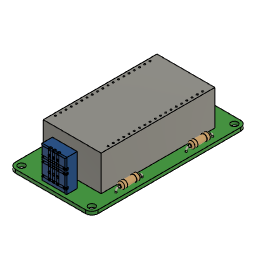
Gr3 3D v1 (Autodesk Fusion 360 archive; units mm, degrees)
design "PCB_PDP"
Autodesk Fusion 360 part; units mm, degrees
note: some values were not read from the file. Set by a fixed rule: which face or edge a step refers to.
sketch "Sketch1" plane through (0, 0, 0) normal (0, 0, 1) x (1, 0, 0)
  line L0 (0, 0) -> (79, 0)
  line L1 (79, 0) -> (79, 44)
  line L2 (79, 44) -> (0, 44)
  line L3 (0, 44) -> (0, 0)
  dimension "d1" = 79
  dimension "d2" = 44
  constraint horizontal L0
  constraint vertical L1
  constraint horizontal L2
  constraint vertical L3
  constraint coincident L0.start L3.end
  measures "d1" distance of L0.start L0.end
  measures "d2" distance of L0.start L2.end
extrude "Extrude1" add sketch "Sketch1" along normal blind 15 makes body 1
shell "Shell1" thickness 1.2 removed faces 1 at (26.3333, 29.3333, 15) on bodies 1
sketch "Sketch7" plane through (0, 0, 1.2) normal (0, 0, 1) x (-1, 0, 0)
  line L0 (-1.2, -42.8) -> (-1.2, -1.2)
  line L1 (-1.2, -1.2) -> (-77.8, -1.2)
  line L2 (-77.8, -1.2) -> (-77.8, -42.8)
  line L3 (-77.8, -42.8) -> (-1.2, -42.8)
  line L4 (-8.3254, -5.15) -> (-6.7377, -7.9)
  line L5 (-6.7377, -7.9) -> (-3.5623, -7.9)
  line L6 (-3.5623, -7.9) -> (-1.9746, -5.15)
  line L7 (-1.9746, -5.15) -> (-3.5623, -2.4)
  line L8 (-3.5623, -2.4) -> (-6.7377, -2.4)
  line L9 (-6.7377, -2.4) -> (-8.3254, -5.15)
  line L10 (-2, -42) -> (-77, -42) construction
  line L11 (-77, -42) -> (-77, -2) construction
  line L12 (-77, -2) -> (-2, -2) construction
  line L13 (-2, -2) -> (-2, -42) construction
  line L14 (-77, -42) -> (-2, -2) construction
  line L15 (-1.2, -42.8) -> (-77.8, -1.2) construction
  line L16 (-7.1996, -8.7) -> (-3.1004, -8.7)
  line L17 (-3.1004, -8.7) -> (-1.0508, -5.15)
  line L18 (-1.0508, -5.15) -> (-3.1004, -1.6)
  line L19 (-3.1004, -1.6) -> (-7.1996, -1.6)
  line L20 (-7.1996, -1.6) -> (-9.2492, -5.15)
  line L21 (-9.2492, -5.15) -> (-7.1996, -8.7)
  circle A0 centre (-5.15, -38.85) radius 3.3
  circle A1 centre (-73.85, -5.15) radius 3.3
  line L22 (-72.2623, -36.1) -> (-75.4377, -36.1)
  line L23 (-75.4377, -36.1) -> (-77.0254, -38.85)
  line L24 (-77.0254, -38.85) -> (-75.4377, -41.6)
  line L25 (-75.4377, -41.6) -> (-72.2623, -41.6)
  line L26 (-72.2623, -41.6) -> (-70.6746, -38.85)
  line L27 (-70.6746, -38.85) -> (-72.2623, -36.1)
  line L28 (-69.7508, -38.85) -> (-71.8004, -35.3)
  line L29 (-71.8004, -35.3) -> (-75.8996, -35.3)
  line L30 (-75.8996, -35.3) -> (-77.9492, -38.85)
  line L31 (-77.9492, -38.85) -> (-75.8996, -42.4)
  line L32 (-75.8996, -42.4) -> (-71.8004, -42.4)
  line L33 (-71.8004, -42.4) -> (-69.7508, -38.85)
  circle A2 centre (-73.85, -38.85) radius 1.55
  circle A3 centre (-5.15, -5.15) radius 1.55
  point P0 (-5.15, -5.15)
  point P1 (-5.15, -5.15)
  point P2 (-73.85, -38.85)
  point P3 (-73.85, -38.85)
  dimension "d63" = 5.5
  dimension "d64" = 75
  dimension "d65" = 40
  dimension "d66" = 3.15
  dimension "d67" = 3.15
  dimension "d68" = 0.8
  dimension "d70" = 3.15
  dimension "d71" = 3.15
  dimension "d72" = 6.6
  dimension "d73" = 6.6
  dimension "d74" = 3.15
  dimension "d75" = 3.15
  dimension "d76" = 5.5
  dimension "d77" = 3.15
  dimension "d78" = 3.15
  dimension "d79" = 0.8
  dimension "d80" = 3.1
  dimension "d81" = 3.1
  constraint horizontal L5
  constraint horizontal L10
  constraint vertical L11
  constraint horizontal L12
  constraint vertical L13
  constraint coincident L0.start L3.end
  constraint coincident L1.end L2.start
  constraint midpoint L14 L15
  constraint coincident P1 P0
  constraint horizontal L16
  constraint horizontal L25
  constraint coincident P3 P2
  constraint horizontal L32
  measures "d63" distance of L6 L9
  measures "d64" distance of L10.start L10.end
  measures "d65" distance of L10.start L12.end
  measures "d66" distance of P1 L12
  measures "d67" distance of P1 L13
  measures "d68" distance of L4 L21
  measures "d70" distance of L10 A0.centre
  measures "d71" distance of L13 A0.centre
  measures "d72" diameter of A0
  measures "d73" diameter of A1
  measures "d74" distance of L12 A1.centre
  measures "d75" distance of L11 A1.centre
  measures "d76" distance of L23 L26
  measures "d77" distance of L10 P3
  measures "d78" distance of L11 P3
  measures "d79" distance of L26 L33
  measures "d80" diameter of A2
  measures "d81" diameter of A3
extrude "Extrude25" cut sketch "Sketch7" against normal blind 4 contours L4 L5 L6 L7 L8 L9 | L22 L23 L24 L25 L26 L27 | A3 bodies 1 makes body 2 at (75.0374, 39.8463, 0.4)
extrude "Extrude26" cut 1 faces at (74.3155, 38.9202, 1.2) along direction (0, 0, -1) blind 7 on bodies 2 bodies 2
extrude "Extrude27" add sketch "Sketch7" along normal blind 1.4 contours L0 L16 L17 L18 L19 L20 L21 | L2 L28 L29 L30 L31 L32 L33 bodies 1 2
extrude "Extrude28" add sketch "Sketch7" along normal blind 3.6 contours A0 | A1 bodies 1
extrude "Extrude29" add sketch "Sketch7" along normal blind 3.6 from surface at 1.4 separate body contours L4 L5 L6 L7 L8 L9 | L22 L23 L24 L25 L26 L27 makes body 3 at (3.6019, 5.2273, 5) makes body 4 at (75.0374, 39.8463, 5)
extrude "Extrude30" add 2 faces at (73.3208, 42.1333, 2.6) (8.2581, 6.3333, 2.6) along direction (0, 0, 1) blind 0.4 on bodies 1 bodies 1 3 4
sketch "Sketch8" plane through (0, 44, 0) normal (0, 1, 0) x (-1, 0, 0)
  line L0 (-79, 0) -> (0, 0)
  line L1 (0, 0) -> (0, 15)
  line L2 (0, 15) -> (-79, 15)
  line L3 (-79, 15) -> (-79, 0)
  line L4 (-76.989, 1.4627) -> (-6.2495, 1.4627) construction
  line L5 (-6.2495, 1.4627) -> (-6.2495, 12.898) construction
  line L6 (-6.2495, 12.898) -> (-76.989, 12.898) construction
  line L7 (-76.989, 12.898) -> (-76.989, 1.4627) construction
  line L8 (-3.0583, 1.7286) -> (-3.0583, 13.6958) construction
  line L9 (-3.0583, 13.6958) -> (-10.7705, 13.6958) construction
  line L10 (-10.7705, 13.6958) -> (-10.7705, 1.7286) construction
  line L11 (-10.7705, 1.7286) -> (-3.0583, 1.7286) construction
  dimension "d114" = 8
  dimension "d115" = 8
  text T0 "TD 2  GR03" font "Arial" height 8 align left top in box 70.7394 x 11.4353 at (-76.989, 1.4627) x (1, 0) y (0, 1) spacing 1 kerned
  text T1 "8>" font "Arial" height 8 align left top in box 11.9672 x 7.7122 at (-3.0583, 1.7286) x (0, 1) y (-1, 0) spacing 1 kerned
extrude "Extrude31" cut sketch "Sketch8" against normal blind 0.4 text T0 T1 bodies 1
extrude "Extrude32" add 1 faces at (8.2581, 6.3333, 3) along direction (0, 0, 1) blind 0.4 on bodies 1 bodies 1
extrude "Extrude33" cut 1 faces at (5.1114, 7.4986, 2.6) along direction (0, 0, 1) blind 0.4 on bodies 1 bodies 1
extrude "Extrude34" add 1 faces at (73.3208, 42.1333, 3) along direction (0, 0, 1) blind 0.4 on bodies 1 bodies 1
extrude "Extrude35" cut 1 faces at (73.8886, 41.1986, 2.6) along direction (0, 0, 1) blind 0.4 on bodies 1 bodies 1
extrude "Extrude36" cut 1 faces at (73.8886, 41.1986, 6.2) along direction (0, 0, -1) blind 1.4 on bodies 1 bodies 1
extrude "Extrude37" cut 1 faces at (5.1114, 7.4986, 6.2) along direction (0, 0, -1) blind 1.4 on bodies 1 bodies 1
extrude "Extrude38" add 1 faces at (5.2123, 2.8038, 3) along direction (0, 0, -1) blind 0.4 on bodies 1 bodies 1
extrude "Extrude39" add 1 faces at (73.9123, 41.1962, 3) along direction (0, 0, -1) blind 0.4 on bodies 1 bodies 1
extrude "Extrude40" cut 1 faces at (26.7333, 43.6, 15) along direction (0, 0, -1) blind 8.6 on bodies 1 bodies 1
extrude "Extrude41" add 1 faces at (52.2667, 0.4, 6.4) along direction (0, 0, 1) blind 0.1 on bodies 1 bodies 1

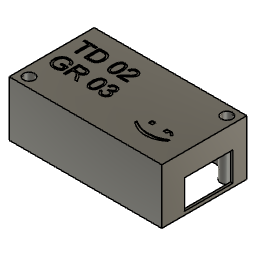
design "Haut"
Autodesk Fusion 360 part; units mm, degrees
sketch "Sketch1" plane through (0, 0, 0) normal (0, 0, 1) x (1, 0, 0)
  line L0 (0, 0) -> (79, 0)
  line L1 (79, 0) -> (79, 44)
  line L2 (79, 44) -> (0, 44)
  line L3 (0, 44) -> (0, 0)
  dimension "d1" = 79
  dimension "d2" = 44
  constraint horizontal L0
  constraint vertical L1
  constraint horizontal L2
  constraint vertical L3
  constraint coincident L0.start L3.end
  measures "d1" distance of L0.start L0.end
  measures "d2" distance of L0.start L2.end
extrude "Extrude1" add sketch "Sketch1" along normal blind 20
shell "Shell1" thickness 1.2 removed faces 1 at (26.3333, 29.3333, 0)
sketch "Sketch2" plane through (0, 0, 18.8) normal (0, 0, -1) x (1, 0, 0)
  line L0 (1.2, -1.2) -> (1.2, -42.8)
  line L1 (1.2, -42.8) -> (77.8, -42.8)
  line L2 (77.8, -42.8) -> (77.8, -1.2)
  line L3 (77.8, -1.2) -> (1.2, -1.2)
  line L4 (1.2, -1.2) -> (77.8, -42.8) construction
  line L5 (2, -2) -> (77, -2)
  line L6 (77, -2) -> (77, -42)
  line L7 (77, -42) -> (2, -42)
  line L8 (2, -42) -> (2, -2)
  line L9 (2, -42) -> (77, -2) construction
  circle A0 centre (5.15, -5.15) radius 1.55
  circle A1 centre (5.15, -5.15) radius 2.9
  circle A2 centre (5.15, -5.15) radius 3.3
  circle A3 centre (73.85, -38.85) radius 1.55
  circle A4 centre (73.85, -38.85) radius 2.9
  circle A5 centre (73.85, -38.85) radius 3.3
  circle A6 centre (5.15, -38.85) radius 2.1
  circle A7 centre (5.15, -38.85) radius 3.3
  circle A8 centre (73.85, -5.15) radius 2.1
  circle A9 centre (73.85, -5.15) radius 3.3
  dimension "d6" = 75
  dimension "d7" = 40
  dimension "d8" = 3.1
  dimension "d9" = 3.15
  dimension "d10" = 5.8
  dimension "d11" = 3.15
  dimension "d12" = 6.6
  dimension "d13" = 3.1
  dimension "d14" = 5.8
  dimension "d15" = 6.6
  dimension "d16" = 3.15
  dimension "d17" = 3.15
  dimension "d18" = 4.2
  dimension "d19" = 6.6
  dimension "d20" = 3.15
  dimension "d21" = 3.15
  dimension "d22" = 4.2
  dimension "d23" = 6.6
  dimension "d24" = 3.15
  dimension "d25" = 3.15
  constraint coincident L0.start L3.end
  constraint coincident L1.end L2.start
  constraint horizontal L5
  constraint vertical L6
  constraint horizontal L7
  constraint vertical L8
  constraint midpoint L4 L9
  constraint concentric A0 A1
  constraint concentric A1 A2
  constraint concentric A3 A4
  constraint concentric A4 A5
  constraint concentric A6 A7
  constraint concentric A8 A9
  measures "d6" distance of L5.start L5.end
  measures "d7" distance of L5.start L7.end
  measures "d8" diameter of A0
  measures "d9" distance of L5 A0.centre
  measures "d10" diameter of A1
  measures "d11" distance of L8 A0.centre
  measures "d12" diameter of A2
  measures "d13" diameter of A3
  measures "d14" diameter of A4
  measures "d15" diameter of A5
  measures "d16" distance of L7 A3.centre
  measures "d17" distance of L6 A3.centre
  measures "d18" diameter of A6
  measures "d19" diameter of A7
  measures "d20" distance of L7 A6.centre
  measures "d21" distance of L8 A6.centre
  measures "d22" diameter of A8
  measures "d23" diameter of A9
  measures "d24" distance of L5 A8.centre
  measures "d25" distance of L6 A8.centre
extrude "Extrude8" cut sketch "Sketch2" against normal blind 3 contours A0 | A1 | A3 | A4
extrude "Extrude9" add sketch "Sketch2" along normal blind 27.4 contours L5 L8 A2 | L5 L6 A9 | L7 L8 A7 | L6 L7 A5 | A1 | A4 picked at (6.3031, -2.2066) picked at (73.7977, -2.352) picked at (5.2023, -41.648) picked at (72.2714, -41.5883)
extrude "Extrude10" cut sketch "Sketch2" along normal blind 22 contours A1 | A4
sketch "Sketch3" plane through (0, 0, 20) normal (0, 0, 1) x (-1, 0, 0)
  circle A0 centre (-5.15, -5.15) radius 2.9
  circle A1 centre (-73.85, -38.85) radius 2.9
  line L0 (0, -44) -> (0, 0)
  line L1 (0, 0) -> (-79, 0)
  line L2 (-79, 0) -> (-79, -44)
  line L3 (-79, -44) -> (0, -44)
  line L4 (-3.2876, -12.007) -> (-62.4651, -12.007) construction
  line L5 (-62.4651, -12.007) -> (-62.4651, -36.0211) construction
  line L6 (-62.4651, -36.0211) -> (-3.2876, -36.0211) construction
  line L7 (-3.2876, -36.0211) -> (-3.2876, -12.007) construction
  dimension "d44" = 8
  text T0 "TD 02\nGR 03" font "Arial" height 8 align left top in box 59.1775 x 24.014 at (-3.2876, -12.007) x (-1, 0) y (0, -1) spacing 1 kerned
extrude "Extrude11" cut sketch "Sketch3" against normal blind 0.4 text T0
sketch "Sketch4" plane through (0, 0, 20) normal (0, 0, 1) x (-1, 0, 0)
  spline S0 degree 3 poles (-14.8865, -28.1575) (-14.6868, -28.1177) (-14.2627, -28.0333) (-13.8303, -28.0253) (-13.6014, -28.0211) knots 0 0 0 0 0.06096 0.129463 0.129463 0.129463 0.129463
  line L0 (-13.6014, -28.0211) -> (-10.7146, -28.0211)
  line L1 (-10.7146, -28.0211) -> (-10.7146, -36.0211)
  line L2 (-10.7146, -36.0211) -> (-13.4704, -36.0211)
  spline S1 degree 3 poles (-13.4704, -36.0211) (-13.7454, -36.0199) (-14.2234, -36.018) (-14.6946, -35.9397) (-14.8947, -35.9065) knots 0 0 0 0 0.082315 0.143089 0.143089 0.143089 0.143089
  spline S2 degree 3 poles (-14.8947, -35.9065) (-15.1133, -35.8449) (-15.5393, -35.7249) (-15.8948, -35.4617) (-16.068, -35.3335) knots 0 0 0 0 0.06748 0.131542 0.131542 0.131542 0.131542
  spline S3 degree 3 poles (-16.068, -35.3335) (-16.2666, -35.1403) (-16.6714, -34.7468) (-16.8989, -34.2298) (-17.0148, -33.9665) knots 0 0 0 0 0.082285 0.167681 0.167681 0.167681 0.167681
  spline S4 degree 3 poles (-17.0148, -33.9665) (-17.1062, -33.6715) (-17.2982, -33.0524) (-17.3181, -32.4041) (-17.3286, -32.0647) knots 0 0 0 0 0.092208 0.193535 0.193535 0.193535 0.193535
  spline S5 degree 3 poles (-17.3286, -32.0647) (-17.3218, -31.7767) (-17.3089, -31.2304) (-17.1778, -30.7002) (-17.1157, -30.4494) knots 0 0 0 0 0.086113 0.16336 0.16336 0.16336 0.16336
  spline S6 degree 3 poles (-17.1157, -30.4494) (-17.0439, -30.2307) (-16.9089, -29.82) (-16.678, -29.455) (-16.57, -29.2844) knots 0 0 0 0 0.068756 0.129091 0.129091 0.129091 0.129091
  spline S7 degree 3 poles (-16.57, -29.2844) (-16.4597, -29.1411) (-16.2487, -28.867) (-15.9731, -28.6582) (-15.8415, -28.5586) knots 0 0 0 0 0.053967 0.103244 0.103244 0.103244 0.103244
  spline S8 degree 3 poles (-15.8415, -28.5586) (-15.6987, -28.4747) (-15.3985, -28.2985) (-15.0626, -28.206) (-14.8865, -28.1575) knots 0 0 0 0 0.049466 0.103977 0.103977 0.103977 0.103977
  spline S9 degree 3 poles (-29.3613, -29.4972) (-29.2824, -29.4107) (-29.1304, -29.244) (-29.0063, -29.0557) (-28.9466, -28.9651) knots 0 0 0 0 0.035063 0.067553 0.067553 0.067553 0.067553
  line L3 (-28.9466, -28.9651) -> (-32.8702, -28.9651)
  line L4 (-32.8702, -28.9651) -> (-32.8702, -28.0211)
  line L5 (-32.8702, -28.0211) -> (-27.5823, -28.0211)
  spline S10 degree 3 poles (-27.5823, -28.0211) (-27.5843, -28.138) (-27.5882, -28.3711) (-27.6608, -28.5927) (-27.6969, -28.7032) knots 0 0 0 0 0.034866 0.069517 0.069517 0.069517 0.069517
  spline S11 degree 3 poles (-27.6969, -28.7032) (-27.7774, -28.8862) (-27.9459, -29.2692) (-28.2071, -29.5964) (-28.3436, -29.7673) knots 0 0 0 0 0.059702 0.124988 0.124988 0.124988 0.124988
  spline S12 degree 3 poles (-28.3436, -29.7673) (-28.5213, -29.9592) (-28.9221, -30.392) (-29.3761, -30.769) (-29.6287, -30.9788) knots 0 0 0 0 0.078394 0.176779 0.176779 0.176779 0.176779
  spline S13 degree 3 poles (-29.6287, -30.9788) (-30.0043, -31.2867) (-30.637, -31.8055) (-31.1733, -32.4224) (-31.3913, -32.6732) knots 0 0 0 0 0.14535 0.24487 0.24487 0.24487 0.24487
  spline S14 degree 3 poles (-31.3913, -32.6732) (-31.5247, -32.8688) (-31.7698, -33.2283) (-31.8247, -33.6585) (-31.8497, -33.8546) knots 0 0 0 0 0.069827 0.128328 0.128328 0.128328 0.128328
  spline S15 degree 3 poles (-31.8497, -33.8546) (-31.8325, -34.0415) (-31.7981, -34.4143) (-31.554, -34.6981) (-31.4322, -34.8396) knots 0 0 0 0 0.054822 0.10938 0.10938 0.10938 0.10938
  spline S16 degree 3 poles (-31.4322, -34.8396) (-31.2782, -34.9566) (-30.957, -35.2005) (-30.5536, -35.2269) (-30.3436, -35.2407) knots 0 0 0 0 0.056724 0.118323 0.118323 0.118323 0.118323
  spline S17 degree 3 poles (-30.3436, -35.2407) (-30.1226, -35.2265) (-29.7, -35.1993) (-29.3672, -34.9391) (-29.2085, -34.8151) knots 0 0 0 0 0.064728 0.123763 0.123763 0.123763 0.123763
  spline S18 degree 3 poles (-29.2085, -34.8151) (-29.0842, -34.6525) (-28.8191, -34.3058) (-28.7919, -33.8686) (-28.7774, -33.6363) knots 0 0 0 0 0.060029 0.128054 0.128054 0.128054 0.128054
  line L6 (-28.7774, -33.6363) -> (-27.7679, -33.74)
  spline S19 degree 3 poles (-27.7679, -33.74) (-27.8182, -34.0867) (-27.9129, -34.7382) (-28.3457, -35.2311) (-28.5482, -35.4617) knots 0 0 0 0 0.10254 0.192668 0.192668 0.192668 0.192668
  spline S20 degree 3 poles (-28.5482, -35.4617) (-28.8041, -35.6342) (-29.3516, -36.0033) (-30.0131, -36.0362) (-30.3654, -36.0538) knots 0 0 0 0 0.090855 0.194374 0.194374 0.194374 0.194374
  spline S21 degree 3 poles (-30.3654, -36.0538) (-30.7214, -36.0342) (-31.393, -35.9973) (-31.9339, -35.6014) (-32.188, -35.4153) knots 0 0 0 0 0.104366 0.196854 0.196854 0.196854 0.196854
  spline S22 degree 3 poles (-32.188, -35.4153) (-32.3838, -35.1889) (-32.7775, -34.7337) (-32.8319, -34.1342) (-32.8593, -33.8328) knots 0 0 0 0 0.087433 0.175808 0.175808 0.175808 0.175808
  spline S23 degree 3 poles (-32.8593, -33.8328) (-32.8507, -33.6725) (-32.8333, -33.3478) (-32.7201, -33.043) (-32.6628, -32.8887) knots 0 0 0 0 0.047865 0.096924 0.096924 0.096924 0.096924
  spline S24 degree 3 poles (-32.6628, -32.8887) (-32.5813, -32.7263) (-32.4045, -32.374) (-32.1486, -32.0738) (-32.0107, -31.9119) knots 0 0 0 0 0.054309 0.117827 0.117827 0.117827 0.117827
  spline S25 degree 3 poles (-32.0107, -31.9119) (-31.8112, -31.7063) (-31.3308, -31.2111) (-30.8043, -30.7649) (-30.4964, -30.504) knots 0 0 0 0 0.085904 0.206877 0.206877 0.206877 0.206877
  spline S26 degree 3 poles (-30.4964, -30.504) (-30.2515, -30.2997) (-29.8628, -29.9756) (-29.4967, -29.6263) (-29.3613, -29.4972) knots 0 0 0 0 0.095636 0.15176 0.15176 0.15176 0.15176
  line L7 (-9.9834, -17.1834) -> (-9.9834, -18.6732)
  line L8 (-9.9834, -18.6732) -> (-7.6314, -18.6732)
  line L9 (-7.6314, -18.6732) -> (-7.6314, -19.6118)
  line L10 (-7.6314, -19.6118) -> (-11.0202, -19.6172)
  line L11 (-11.0202, -19.6172) -> (-11.0202, -16.6486)
  spline S27 degree 3 poles (-11.0202, -16.6486) (-10.7625, -16.4558) (-10.262, -16.0814) (-9.6885, -15.8331) (-9.4104, -15.7127) knots 0 0 0 0 0.096193 0.186779 0.186779 0.186779 0.186779
  spline S28 degree 3 poles (-9.4104, -15.7127) (-9.1327, -15.6212) (-8.5795, -15.4389) (-7.9976, -15.4122) (-7.7078, -15.399) knots 0 0 0 0 0.087271 0.173848 0.173848 0.173848 0.173848
  spline S29 degree 3 poles (-7.7078, -15.399) (-7.3274, -15.4182) (-6.5823, -15.4558) (-5.9, -15.7565) (-5.5659, -15.9037) knots 0 0 0 0 0.113189 0.221711 0.221711 0.221711 0.221711
  spline S30 degree 3 poles (-5.5659, -15.9037) (-5.2648, -16.0902) (-4.6646, -16.4619) (-4.2956, -17.0636) (-4.1116, -17.3635) knots 0 0 0 0 0.10466 0.208619 0.208619 0.208619 0.208619
  spline S31 degree 3 poles (-4.1116, -17.3635) (-3.9684, -17.6957) (-3.6749, -18.3766) (-3.6389, -19.1177) (-3.6205, -19.4972) knots 0 0 0 0 0.107593 0.220541 0.220541 0.220541 0.220541
  spline S32 degree 3 poles (-3.6205, -19.4972) (-3.64, -19.8783) (-3.6787, -20.6329) (-3.9665, -21.3315) (-4.1089, -21.6773) knots 0 0 0 0 0.113551 0.224866 0.224866 0.224866 0.224866
  spline S33 degree 3 poles (-4.1089, -21.6773) (-4.2863, -21.9912) (-4.6337, -22.6062) (-5.2247, -22.9919) (-5.5141, -23.1807) knots 0 0 0 0 0.10642 0.208487 0.208487 0.208487 0.208487
  spline S34 degree 3 poles (-5.5141, -23.1807) (-5.838, -23.3239) (-6.5103, -23.6211) (-7.2452, -23.6545) (-7.626, -23.6718) knots 0 0 0 0 0.105289 0.218508 0.218508 0.218508 0.218508
  spline S35 degree 3 poles (-7.626, -23.6718) (-7.9038, -23.6619) (-8.4403, -23.6426) (-8.9494, -23.4727) (-9.1949, -23.3908) knots 0 0 0 0 0.082904 0.16012 0.16012 0.16012 0.16012
  spline S36 degree 3 poles (-9.1949, -23.3908) (-9.4128, -23.2918) (-9.8307, -23.102) (-10.1444, -22.7677) (-10.2945, -22.6077) knots 0 0 0 0 0.071018 0.136162 0.136162 0.136162 0.136162
  spline S37 degree 3 poles (-10.2945, -22.6077) (-10.4213, -22.4196) (-10.6932, -22.016) (-10.8282, -21.5479) (-10.9002, -21.298) knots 0 0 0 0 0.067641 0.145087 0.145087 0.145087 0.145087
  line L12 (-10.9002, -21.298) -> (-9.9452, -21.0361)
  spline S38 degree 3 poles (-9.9452, -21.0361) (-9.8865, -21.2221) (-9.7792, -21.5622) (-9.5855, -21.8611) (-9.4977, -21.9965) knots 0 0 0 0 0.058186 0.106384 0.106384 0.106384 0.106384
  spline S39 degree 3 poles (-9.4977, -21.9965) (-9.395, -22.1088) (-9.1781, -22.346) (-8.887, -22.4834) (-8.7337, -22.5559) knots 0 0 0 0 0.045201 0.095494 0.095494 0.095494 0.095494
  spline S40 degree 3 poles (-8.7337, -22.5559) (-8.5608, -22.6171) (-8.2043, -22.7434) (-7.8262, -22.7583) (-7.6314, -22.766) knots 0 0 0 0 0.054706 0.112788 0.112788 0.112788 0.112788
  spline S41 degree 3 poles (-7.6314, -22.766) (-7.4038, -22.7592) (-6.9743, -22.7464) (-6.5675, -22.6093) (-6.3763, -22.5449) knots 0 0 0 0 0.067892 0.128065 0.128065 0.128065 0.128065
  spline S42 degree 3 poles (-6.3763, -22.5449) (-6.211, -22.4683) (-5.8941, -22.3214) (-5.6426, -22.0795) (-5.5223, -21.9638) knots 0 0 0 0 0.054229 0.103942 0.103942 0.103942 0.103942
  spline S43 degree 3 poles (-5.5223, -21.9638) (-5.4204, -21.8415) (-5.2185, -21.5991) (-5.0841, -21.3138) (-5.0175, -21.1725) knots 0 0 0 0 0.047546 0.094197 0.094197 0.094197 0.094197
  spline S44 degree 3 poles (-5.0175, -21.1725) (-4.9284, -20.9171) (-4.7465, -20.3958) (-4.7236, -19.8441) (-4.7119, -19.5627) knots 0 0 0 0 0.080677 0.164655 0.164655 0.164655 0.164655
  spline S45 degree 3 poles (-4.7119, -19.5627) (-4.7223, -19.2309) (-4.7417, -18.6121) (-4.973, -18.0387) (-5.0803, -17.7728) knots 0 0 0 0 0.098657 0.184016 0.184016 0.184016 0.184016
  spline S46 degree 3 poles (-5.0803, -17.7728) (-5.2161, -17.5486) (-5.4856, -17.1037) (-5.9314, -16.836) (-6.1526, -16.7032) knots 0 0 0 0 0.077354 0.153502 0.153502 0.153502 0.153502
  spline S47 degree 3 poles (-6.1526, -16.7032) (-6.3911, -16.6013) (-6.869, -16.3972) (-7.3879, -16.3684) (-7.6478, -16.3539) knots 0 0 0 0 0.07716 0.154598 0.154598 0.154598 0.154598
  spline S48 degree 3 poles (-7.6478, -16.3539) (-7.8764, -16.3653) (-8.3367, -16.3881) (-8.7714, -16.5414) (-8.9902, -16.6186) knots 0 0 0 0 0.068261 0.137472 0.137472 0.137472 0.137472
  spline S49 degree 3 poles (-8.9902, -16.6186) (-9.187, -16.7013) (-9.541, -16.8501) (-9.8474, -17.0809) (-9.9834, -17.1834) knots 0 0 0 0 0.063739 0.114642 0.114642 0.114642 0.114642
  spline S50 degree 3 poles (-25.967, -15.399) (-25.6051, -15.4299) (-24.8991, -15.4902) (-24.3953, -15.9865) (-24.1498, -16.2284) knots 0 0 0 0 0.105336 0.205454 0.205454 0.205454 0.205454
  spline S51 degree 3 poles (-24.1498, -16.2284) (-23.9204, -16.6574) (-23.3802, -17.667) (-23.3665, -18.8185) (-23.3586, -19.4808) knots 0 0 0 0 0.144035 0.339038 0.339038 0.339038 0.339038
  spline S52 degree 3 poles (-23.3586, -19.4808) (-23.3644, -19.9101) (-23.3748, -20.6833) (-23.5656, -21.4317) (-23.6505, -21.7646) knots 0 0 0 0 0.128243 0.230946 0.230946 0.230946 0.230946
  spline S53 degree 3 poles (-23.6505, -21.7646) (-23.7539, -22.0316) (-23.95, -22.5379) (-24.3358, -22.9188) (-24.5182, -23.0988) knots 0 0 0 0 0.084764 0.160768 0.160768 0.160768 0.160768
  spline S54 degree 3 poles (-24.5182, -23.0988) (-24.7284, -23.2356) (-25.1682, -23.5219) (-25.6931, -23.5523) (-25.967, -23.5681) knots 0 0 0 0 0.073924 0.154658 0.154658 0.154658 0.154658
  spline S55 degree 3 poles (-25.967, -23.5681) (-26.1715, -23.5592) (-26.5643, -23.5421) (-26.9241, -23.3845) (-27.0966, -23.3089) knots 0 0 0 0 0.060783 0.116789 0.116789 0.116789 0.116789
  spline S56 degree 3 poles (-27.0966, -23.3089) (-27.2522, -23.2118) (-27.568, -23.0147) (-27.7875, -22.7139) (-27.8988, -22.5613) knots 0 0 0 0 0.054476 0.110564 0.110564 0.110564 0.110564
  spline S57 degree 3 poles (-27.8988, -22.5613) (-28.0001, -22.3838) (-28.2145, -22.0079) (-28.3329, -21.5915) (-28.3954, -21.3717) knots 0 0 0 0 0.061081 0.129332 0.129332 0.129332 0.129332
  spline S58 degree 3 poles (-28.3954, -21.3717) (-28.4477, -21.098) (-28.5671, -20.4738) (-28.5725, -19.8379) (-28.5755, -19.4808) knots 0 0 0 0 0.083433 0.190281 0.190281 0.190281 0.190281
  spline S59 degree 3 poles (-28.5755, -19.4808) (-28.5697, -19.0543) (-28.5591, -18.285) (-28.3704, -17.5399) (-28.2863, -17.208) knots 0 0 0 0 0.127422 0.229814 0.229814 0.229814 0.229814
  spline S60 degree 3 poles (-28.2863, -17.208) (-28.1836, -16.9408) (-27.9887, -16.4337) (-27.6036, -16.0517) (-27.4213, -15.871) knots 0 0 0 0 0.084738 0.16085 0.16085 0.16085 0.16085
  spline S61 degree 3 poles (-27.4213, -15.871) (-27.2107, -15.7334) (-26.7696, -15.4452) (-26.2425, -15.4148) (-25.967, -15.399) knots 0 0 0 0 0.074142 0.155291 0.155291 0.155291 0.155291
  line L13 (-13.656, -19.0879) -> (-13.656, -15.5354)
  line L14 (-13.656, -15.5354) -> (-12.5973, -15.5354)
  line L15 (-12.5973, -15.5354) -> (-12.5973, -23.5354)
  line L16 (-12.5973, -23.5354) -> (-16.1444, -23.5354)
  spline S62 degree 3 poles (-16.1444, -23.5354) (-16.4604, -23.533) (-17.0123, -23.5287) (-17.5436, -23.3824) (-17.7706, -23.3198) knots 0 0 0 0 0.094288 0.164656 0.164656 0.164656 0.164656
  spline S63 degree 3 poles (-17.7706, -23.3198) (-17.9478, -23.2326) (-18.3089, -23.0548) (-18.5416, -22.726) (-18.6601, -22.5586) knots 0 0 0 0 0.05827 0.118743 0.118743 0.118743 0.118743
  spline S64 degree 3 poles (-18.6601, -22.5586) (-18.7572, -22.371) (-18.953, -21.9925) (-18.9796, -21.5671) (-18.993, -21.3526) knots 0 0 0 0 0.062627 0.126338 0.126338 0.126338 0.126338
  spline S65 degree 3 poles (-18.993, -21.3526) (-18.9715, -21.0816) (-18.9293, -20.5483) (-18.6025, -20.1254) (-18.4418, -19.9174) knots 0 0 0 0 0.079646 0.15674 0.15674 0.15674 0.15674
  spline S66 degree 3 poles (-18.4418, -19.9174) (-18.217, -19.7387) (-17.7177, -19.3417) (-17.0863, -19.2343) (-16.7392, -19.1752) knots 0 0 0 0 0.084836 0.188411 0.188411 0.188411 0.188411
  spline S67 degree 3 poles (-16.7392, -19.1752) (-16.8653, -19.1129) (-17.0915, -19.0012) (-17.2899, -18.8457) (-17.3777, -18.7769) knots 0 0 0 0 0.04206 0.075431 0.075431 0.075431 0.075431
  spline S68 degree 3 poles (-17.3777, -18.7769) (-17.5332, -18.6214) (-17.8601, -18.2949) (-18.12, -17.9129) (-18.2563, -17.7127) knots 0 0 0 0 0.065819 0.138268 0.138268 0.138268 0.138268
  line L17 (-18.2563, -17.7127) -> (-19.6478, -15.5354)
  line L18 (-19.6478, -15.5354) -> (-18.3163, -15.5354)
  line L19 (-18.3163, -15.5354) -> (-17.2576, -17.1998)
  spline S69 degree 3 poles (-17.2576, -17.1998) (-17.1193, -17.4135) (-16.8762, -17.7891) (-16.6088, -18.1476) (-16.4936, -18.3021) knots 0 0 0 0 0.076356 0.134151 0.134151 0.134151 0.134151
  spline S70 degree 3 poles (-16.4936, -18.3021) (-16.4033, -18.415) (-16.2442, -18.6138) (-16.0431, -18.7695) (-15.9561, -18.8369) knots 0 0 0 0 0.043167 0.076058 0.076058 0.076058 0.076058
  spline S71 degree 3 poles (-15.9561, -18.8369) (-15.8779, -18.8837) (-15.7257, -18.9746) (-15.5557, -19.0252) (-15.4732, -19.0497) knots 0 0 0 0 0.027225 0.05296 0.05296 0.05296 0.05296
  spline S72 degree 3 poles (-15.4732, -19.0497) (-15.3942, -19.0608) (-15.1988, -19.0881) (-15.0014, -19.088) (-14.8838, -19.0879) knots 0 0 0 0 0.02391 0.059121 0.059121 0.059121 0.059121
  line L20 (-14.8838, -19.0879) -> (-13.656, -19.0879)
  spline S73 degree 3 poles (-32.1226, -15.3935) (-31.7904, -15.4161) (-31.1469, -15.4599) (-30.6257, -15.8381) (-30.3736, -16.0211) knots 0 0 0 0 0.097653 0.189193 0.189193 0.189193 0.189193
  spline S74 degree 3 poles (-30.3736, -16.0211) (-30.1663, -16.2488) (-29.7436, -16.713) (-29.635, -17.3319) (-29.5796, -17.6473) knots 0 0 0 0 0.090411 0.184321 0.184321 0.184321 0.184321
  line L21 (-29.5796, -17.6473) -> (-30.5619, -17.7782)
  spline S75 degree 3 poles (-30.5619, -17.7782) (-30.6185, -17.529) (-30.7199, -17.0825) (-31.0096, -16.7305) (-31.1376, -16.575) knots 0 0 0 0 0.075375 0.135022 0.135022 0.135022 0.135022
  spline S76 degree 3 poles (-31.1376, -16.575) (-31.2821, -16.4675) (-31.5762, -16.2489) (-31.942, -16.2209) (-32.128, -16.2066) knots 0 0 0 0 0.052879 0.107615 0.107615 0.107615 0.107615
  spline S77 degree 3 poles (-32.128, -16.2066) (-32.3495, -16.2261) (-32.7897, -16.2648) (-33.1297, -16.5468) (-33.2985, -16.6868) knots 0 0 0 0 0.065033 0.129227 0.129227 0.129227 0.129227
  spline S78 degree 3 poles (-33.2985, -16.6868) (-33.4378, -16.858) (-33.72, -17.2047) (-33.7572, -17.6506) (-33.776, -17.8765) knots 0 0 0 0 0.064589 0.130884 0.130884 0.130884 0.130884
  spline S79 degree 3 poles (-33.776, -17.8765) (-33.7594, -18.0903) (-33.7268, -18.5084) (-33.4629, -18.8336) (-33.334, -18.9924) knots 0 0 0 0 0.062714 0.122592 0.122592 0.122592 0.122592
  spline S80 degree 3 poles (-33.334, -18.9924) (-33.1739, -19.1205) (-32.8454, -19.3834) (-32.4253, -19.4153) (-32.2099, -19.4317) knots 0 0 0 0 0.06005 0.123222 0.123222 0.123222 0.123222
  spline S81 degree 3 poles (-32.2099, -19.4317) (-32.1053, -19.4255) (-31.8709, -19.4115) (-31.643, -19.3543) (-31.5168, -19.3226) knots 0 0 0 0 0.031361 0.070293 0.070293 0.070293 0.070293
  line L22 (-31.5168, -19.3226) -> (-31.626, -20.1848)
  spline S82 degree 3 poles (-31.626, -20.1848) (-31.6555, -20.1816) (-31.7081, -20.176) (-31.761, -20.1745) (-31.7842, -20.1739) knots 0 0 0 0 0.008905 0.015868 0.015868 0.015868 0.015868
  spline S83 degree 3 poles (-31.7842, -20.1739) (-31.9871, -20.1868) (-32.388, -20.2124) (-32.74, -20.4058) (-32.9138, -20.5013) knots 0 0 0 0 0.060178 0.118901 0.118901 0.118901 0.118901
  spline S84 degree 3 poles (-32.9138, -20.5013) (-33.0602, -20.6293) (-33.3648, -20.8958) (-33.3984, -21.3006) (-33.4159, -21.5108) knots 0 0 0 0 0.056117 0.116775 0.116775 0.116775 0.116775
  spline S85 degree 3 poles (-33.4159, -21.5108) (-33.4017, -21.6822) (-33.3737, -22.0192) (-33.1569, -22.2784) (-33.0503, -22.4058) knots 0 0 0 0 0.050225 0.098812 0.098812 0.098812 0.098812
  spline S86 degree 3 poles (-33.0503, -22.4058) (-32.9163, -22.5092) (-32.6386, -22.7237) (-32.2878, -22.7479) (-32.1062, -22.7605) knots 0 0 0 0 0.049617 0.102885 0.102885 0.102885 0.102885
  spline S87 degree 3 poles (-32.1062, -22.7605) (-31.9248, -22.747) (-31.5706, -22.7207) (-31.2887, -22.5054) (-31.1512, -22.4003) knots 0 0 0 0 0.05329 0.104049 0.104049 0.104049 0.104049
  spline S88 degree 3 poles (-31.1512, -22.4003) (-31.0341, -22.2562) (-30.7772, -21.9401) (-30.7013, -21.5384) (-30.6601, -21.3198) knots 0 0 0 0 0.054876 0.120353 0.120353 0.120353 0.120353
  line L23 (-30.6601, -21.3198) -> (-29.6778, -21.4945)
  spline S89 degree 3 poles (-29.6778, -21.4945) (-29.7513, -21.8002) (-29.8913, -22.3829) (-30.3014, -22.8182) (-30.4964, -23.0252) knots 0 0 0 0 0.092474 0.176282 0.176282 0.176282 0.176282
  spline S90 degree 3 poles (-30.4964, -23.0252) (-30.7272, -23.1835) (-31.2053, -23.5113) (-31.7847, -23.5488) (-32.0844, -23.5681) knots 0 0 0 0 0.082391 0.170618 0.170618 0.170618 0.170618
  spline S91 degree 3 poles (-32.0844, -23.5681) (-32.2969, -23.5571) (-32.7158, -23.5355) (-33.1008, -23.3691) (-33.2904, -23.2871) knots 0 0 0 0 0.063283 0.12472 0.12472 0.12472 0.12472
  spline S92 degree 3 poles (-33.2904, -23.2871) (-33.4621, -23.1869) (-33.7977, -22.9909) (-34.0233, -22.6748) (-34.1335, -22.5204) knots 0 0 0 0 0.058898 0.115119 0.115119 0.115119 0.115119
  spline S93 degree 3 poles (-34.1335, -22.5204) (-34.2186, -22.3569) (-34.3872, -22.0332) (-34.4128, -21.6692) (-34.4254, -21.489) knots 0 0 0 0 0.054647 0.108216 0.108216 0.108216 0.108216
  spline S94 degree 3 poles (-34.4254, -21.489) (-34.4141, -21.3204) (-34.3915, -20.985) (-34.2283, -20.6911) (-34.1471, -20.5449) knots 0 0 0 0 0.050009 0.099509 0.099509 0.099509 0.099509
  spline S95 degree 3 poles (-34.1471, -20.5449) (-34.0395, -20.4087) (-33.8143, -20.1236) (-33.4916, -19.9558) (-33.3231, -19.8683) knots 0 0 0 0 0.051483 0.107709 0.107709 0.107709 0.107709
  spline S96 degree 3 poles (-33.3231, -19.8683) (-33.5441, -19.8019) (-33.9727, -19.6733) (-34.2777, -19.3469) (-34.4254, -19.1889) knots 0 0 0 0 0.067869 0.131566 0.131566 0.131566 0.131566
  spline S97 degree 3 poles (-34.4254, -19.1889) (-34.5399, -19.0005) (-34.7806, -18.6046) (-34.8054, -18.1412) (-34.8183, -17.8983) knots 0 0 0 0 0.0651 0.136786 0.136786 0.136786 0.136786
  spline S98 degree 3 poles (-34.8183, -17.8983) (-34.7862, -17.5621) (-34.7219, -16.8882) (-34.2772, -16.3778) (-34.0543, -16.122) knots 0 0 0 0 0.098661 0.197741 0.197741 0.197741 0.197741
  spline S99 degree 3 poles (-34.0543, -16.122) (-33.7777, -15.9096) (-33.2083, -15.4724) (-32.4912, -15.4203) (-32.1226, -15.3935) knots 0 0 0 0 0.102306 0.210534 0.210534 0.210534 0.210534
  spline S100 degree 3 poles (-24.1007, -27.8846) (-23.7388, -27.9156) (-23.0327, -27.9759) (-22.529, -28.4722) (-22.2835, -28.7141) knots 0 0 0 0 0.105336 0.205454 0.205454 0.205454 0.205454
  spline S101 degree 3 poles (-22.2835, -28.7141) (-22.0541, -29.143) (-21.5139, -30.1527) (-21.5002, -31.3042) (-21.4923, -31.9665) knots 0 0 0 0 0.144035 0.339039 0.339039 0.339039 0.339039
  spline S102 degree 3 poles (-21.4923, -31.9665) (-21.4981, -32.3958) (-21.5085, -33.169) (-21.6993, -33.9174) (-21.7842, -34.2503) knots 0 0 0 0 0.128243 0.230946 0.230946 0.230946 0.230946
  spline S103 degree 3 poles (-21.7842, -34.2503) (-21.8876, -34.5172) (-22.0837, -35.0236) (-22.4695, -35.4044) (-22.6519, -35.5845) knots 0 0 0 0 0.084764 0.160768 0.160768 0.160768 0.160768
  spline S104 degree 3 poles (-22.6519, -35.5845) (-22.8621, -35.7213) (-23.3019, -36.0075) (-23.8267, -36.0379) (-24.1007, -36.0538) knots 0 0 0 0 0.073924 0.154658 0.154658 0.154658 0.154658
  spline S105 degree 3 poles (-24.1007, -36.0538) (-24.3052, -36.0449) (-24.698, -36.0277) (-25.0578, -35.8702) (-25.2303, -35.7946) knots 0 0 0 0 0.060783 0.116789 0.116789 0.116789 0.116789
  spline S106 degree 3 poles (-25.2303, -35.7946) (-25.3859, -35.6975) (-25.7017, -35.5004) (-25.9212, -35.1996) (-26.0325, -35.047) knots 0 0 0 0 0.054476 0.110564 0.110564 0.110564 0.110564
  spline S107 degree 3 poles (-26.0325, -35.047) (-26.1338, -34.8695) (-26.3482, -34.4936) (-26.4666, -34.0771) (-26.5291, -33.8574) knots 0 0 0 0 0.061081 0.129331 0.129331 0.129331 0.129331
  spline S108 degree 3 poles (-26.5291, -33.8574) (-26.5814, -33.5837) (-26.7008, -32.9595) (-26.7062, -32.3236) (-26.7092, -31.9665) knots 0 0 0 0 0.083433 0.190281 0.190281 0.190281 0.190281
  spline S109 degree 3 poles (-26.7092, -31.9665) (-26.7034, -31.54) (-26.6928, -30.7707) (-26.5041, -30.0256) (-26.42, -29.6936) knots 0 0 0 0 0.127422 0.229814 0.229814 0.229814 0.229814
  spline S110 degree 3 poles (-26.42, -29.6936) (-26.3173, -29.4265) (-26.1224, -28.9194) (-25.7373, -28.5374) (-25.555, -28.3567) knots 0 0 0 0 0.084738 0.16085 0.16085 0.16085 0.16085
  spline S111 degree 3 poles (-25.555, -28.3567) (-25.3444, -28.2191) (-24.9033, -27.9309) (-24.3762, -27.9005) (-24.1007, -27.8846) knots 0 0 0 0 0.074141 0.155291 0.155291 0.155291 0.155291
  line L24 (-6.982, -35.077) -> (-6.982, -28.0211)
  line L25 (-6.982, -28.0211) -> (-5.9234, -28.0211)
  line L26 (-5.9234, -28.0211) -> (-5.9234, -35.077)
  line L27 (-5.9234, -35.077) -> (-3.2876, -35.077)
  line L28 (-3.2876, -35.077) -> (-3.2876, -36.0211)
  line L29 (-3.2876, -36.0211) -> (-9.6287, -36.0211)
  line L30 (-9.6287, -36.0211) -> (-9.6287, -35.077)
  line L31 (-9.6287, -35.077) -> (-6.982, -35.077)
  circle A0 centre (-5.15, -5.15) radius 2.9
  circle A1 centre (-73.85, -38.85) radius 2.9
  line L32 (0, -44) -> (0, 0)
  line L33 (0, 0) -> (-79, 0)
  line L34 (-79, 0) -> (-79, -44)
  line L35 (-79, -44) -> (0, -44)
  line L36 (-71.0312, -8.9144) -> (-71.0415, -20.7264) construction
  line L37 (-71.0415, -20.7264) -> (-53.1263, -20.7421) construction
  line L38 (-53.1263, -20.7421) -> (-53.116, -8.9301) construction
  line L39 (-53.116, -8.9301) -> (-71.0312, -8.9144) construction
  dimension "d48" = 13
  text T0 "(;" font "Arial" height 13 align left top in box 11.812 x 17.9152 at (-71.0312, -8.9144) x (-0.000873, -1) y (1, -0.000873) spacing 1 kerned
extrude "Extrude12" add sketch "Sketch4" along normal blind 0.4 text T0
extrude "Extrude15" add 1 faces at (26.7333, 43.6, 0) along direction (0, 0, -1) blind 8.6
extrude "Extrude16" cut 3 faces at (63.524, 10.2844, 20.4) (57.9167, 16.0939, 20.4) (64.9106, 16.3893, 20.4) along direction (0, 0, -1) blind 0.8
extrude "Extrude13" add 2 faces at (7.5892, 5.2941, -3.2) (74.2523, 41.2601, -3.2) along direction (0, 0, 1) blind 0.4
sketch "Sketch5" plane through (79, 0, 0) normal (1, 0, 0) x (0, 1, 0)
  line L0 (44, -8.6) -> (44, 20)
  line L1 (44, 20) -> (0, 20)
  line L2 (0, 20) -> (0, -8.6)
  line L3 (11.8, 8.3) -> (36.8, 8.3)
  line L4 (36.8, 8.3) -> (36.8, -6.7)
  line L5 (36.8, -6.7) -> (11.8, -6.7)
  line L6 (11.8, -6.7) -> (11.8, 8.3)
  line L7 (0, -8.6) -> (44, -8.6)
  line L8 (11.8, 8.3) -> (36.8, -6.7) construction
  dimension "d53" = 25
  dimension "d54" = 15
  dimension "d61" = 1.9
  dimension "d62" = 7.2
  constraint horizontal L3
  constraint vertical L4
  constraint horizontal L5
  constraint vertical L6
  measures "d53" distance of L3.start L3.end
  measures "d54" distance of L3.start L5.end
  measures "d61" distance of L5.end L7
  measures "d62" distance of L0 L4
extrude "Extrude17" cut sketch "Sketch5" against normal blind 1.2 contours L3 L4 L5 L6
extrude "Extrude18" cut 5 faces at (73.7877, 41.4629, -8.6) (26.7333, 43.6, -8.6) (73.7977, 2.352, -8.6) (5.2123, 2.5371, -8.6) (5.2344, 41.6449, -8.6) along direction (0, 0, 1) blind 0.1
sketch "Sketch6" plane through (0, 0, 0) normal (-1, 0, 0) x (0, -1, 0)
  line L0 (-44, -8.5) -> (0, -8.5)
  line L1 (0, -8.5) -> (0, 20)
  line L2 (0, 20) -> (-44, 20)
  line L3 (-44, 20) -> (-44, -8.5)
  line L4 (-26.4, -5.5) -> (-25.2, -5.5)
  line L5 (-25.2, -5.5) -> (-25.2, -4.3)
  line L6 (-25.2, -4.3) -> (-26.4, -4.3)
  line L7 (-26.4, -4.3) -> (-26.4, -5.5)
  line L8 (-24, -4.3) -> (-22.8, -4.3)
  line L9 (-22.8, -4.3) -> (-22.8, -5.5)
  line L10 (-22.8, -5.5) -> (-24, -5.5)
  line L11 (-24, -5.5) -> (-24, -4.3)
  line L12 (-21.6, -1.9) -> (-20.4, -1.9)
  line L13 (-20.4, -1.9) -> (-20.4, -3.1)
  line L14 (-20.4, -3.1) -> (-21.6, -3.1)
  line L15 (-21.6, -3.1) -> (-21.6, -1.9)
  line L16 (-24, -1.9) -> (-22.8, -1.9)
  line L17 (-22.8, -1.9) -> (-22.8, -3.1)
  line L18 (-22.8, -3.1) -> (-24, -3.1)
  line L19 (-24, -3.1) -> (-24, -1.9)
  line L20 (-21.6, -4.3) -> (-20.4, -4.3)
  line L21 (-20.4, -4.3) -> (-20.4, -5.5)
  line L22 (-20.4, -5.5) -> (-21.6, -5.5)
  line L23 (-21.6, -5.5) -> (-21.6, -4.3)
  line L24 (-26.4, -1.9) -> (-25.2, -1.9)
  line L25 (-25.2, -1.9) -> (-25.2, -3.1)
  line L26 (-25.2, -3.1) -> (-26.4, -3.1)
  line L27 (-26.4, -3.1) -> (-26.4, -1.9)
  line L28 (-26.4, 0.5) -> (-25.2, 0.5)
  line L29 (-25.2, 0.5) -> (-25.2, -0.7)
  line L30 (-25.2, -0.7) -> (-26.4, -0.7)
  line L31 (-26.4, -0.7) -> (-26.4, 0.5)
  line L32 (-19.2, -4.3) -> (-18, -4.3)
  line L33 (-18, -4.3) -> (-18, -5.5)
  line L34 (-18, -5.5) -> (-19.2, -5.5)
  line L35 (-19.2, -5.5) -> (-19.2, -4.3)
  line L36 (-24, 0.5) -> (-22.8, 0.5)
  line L37 (-22.8, 0.5) -> (-22.8, -0.7)
  line L38 (-22.8, -0.7) -> (-24, -0.7)
  line L39 (-24, -0.7) -> (-24, 0.5)
  line L40 (-21.6, 0.5) -> (-20.4, 0.5)
  line L41 (-20.4, 0.5) -> (-20.4, -0.7)
  line L42 (-20.4, -0.7) -> (-21.6, -0.7)
  line L43 (-21.6, -0.7) -> (-21.6, 0.5)
  line L44 (-19.2, -1.9) -> (-18, -1.9)
  line L45 (-18, -1.9) -> (-18, -3.1)
  line L46 (-18, -3.1) -> (-19.2, -3.1)
  line L47 (-19.2, -3.1) -> (-19.2, -1.9)
  line L48 (-19.2, 0.5) -> (-18, 0.5)
  line L49 (-18, 0.5) -> (-18, -0.7)
  line L50 (-18, -0.7) -> (-19.2, -0.7)
  line L51 (-19.2, -0.7) -> (-19.2, 0.5)
  line L52 (-18, 0.5) -> (-26.4, 0.5) construction
  dimension "d67" = 1.2
  dimension "d68" = 1.2
  dimension "d69" = 3
  dimension "d70" = 17.6
  dimension "d71" = 1.2
  dimension "d72" = 1.2
  dimension "d73" = 1.2
  dimension "d74" = 1.2
  dimension "d75" = 1.2
  dimension "d76" = 1.2
  dimension "d77" = 1.2
  dimension "d78" = 1.2
  dimension "d79" = 1.2
  dimension "d80" = 1.2
  dimension "d81" = 3
  dimension "d82" = 1.2
  dimension "d83" = 3
  dimension "d84" = 1.2
  dimension "d85" = 1.2
  dimension "d86" = 1.2
  dimension "d87" = 1.2
  dimension "d88" = 1.2
  dimension "d89" = 1.2
  dimension "d90" = 17.6
  dimension "d91" = 1.2
  dimension "d92" = 1.2
  dimension "d93" = 1.2
  dimension "d94" = 1.2
  dimension "d95" = 1.2
  dimension "d96" = 1.2
  dimension "d97" = 1.2
  dimension "d98" = 1.2
  dimension "d99" = 17.6
  dimension "d100" = 1.2
  dimension "d101" = 1.2
  dimension "d102" = 1.2
  dimension "d103" = 1.2
  dimension "d104" = 1.2
  dimension "d105" = 1.2
  dimension "d106" = 3
  dimension "d107" = 1.2
  dimension "d108" = 1.2
  dimension "d109" = 1.2
  dimension "d110" = 1.2
  dimension "d111" = 1.2
  dimension "d112" = 1.2
  dimension "d115" = 1.2
  dimension "d116" = 1.2
  constraint horizontal L4
  constraint vertical L5
  constraint horizontal L6
  constraint vertical L7
  constraint horizontal L8
  constraint vertical L9
  constraint horizontal L10
  constraint vertical L11
  constraint horizontal L12
  constraint vertical L13
  constraint horizontal L14
  constraint vertical L15
  constraint horizontal L16
  constraint vertical L17
  constraint horizontal L18
  constraint vertical L19
  constraint horizontal L20
  constraint vertical L21
  constraint horizontal L22
  constraint vertical L23
  constraint horizontal L24
  constraint vertical L25
  constraint horizontal L26
  constraint vertical L27
  constraint horizontal L28
  constraint vertical L29
  constraint horizontal L30
  constraint vertical L31
  constraint horizontal L32
  constraint vertical L33
  constraint horizontal L34
  constraint vertical L35
  constraint horizontal L36
  constraint vertical L37
  constraint horizontal L38
  constraint vertical L39
  constraint horizontal L40
  constraint vertical L41
  constraint horizontal L42
  constraint vertical L43
  constraint horizontal L44
  constraint vertical L45
  constraint horizontal L46
  constraint vertical L47
  constraint horizontal L48
  constraint vertical L49
  constraint horizontal L50
  constraint vertical L51
  measures "d67" distance of L4.start L4.end
  measures "d68" distance of L4.start L6.end
  measures "d69" distance of L0 L4
  measures "d70" distance of L3 L7
  measures "d71" distance of L8.start L8.end
  measures "d72" distance of L8.start L10.end
  measures "d73" distance of L12.start L12.end
  measures "d74" distance of L12.start L14.end
  measures "d75" distance of L16.start L16.end
  measures "d76" distance of L16.start L18.end
  measures "d77" distance of L20.start L20.end
  measures "d78" distance of L20.start L22.end
  measures "d79" distance of L24.start L24.end
  measures "d80" distance of L24.start L26.end
  measures "d81" distance of L0 L10
  measures "d82" distance of L5 L11
  measures "d83" distance of L0 L22
  measures "d84" distance of L9 L23
  measures "d85" distance of L6 L26
  measures "d86" distance of L8 L18
  measures "d87" distance of L19 L25
  measures "d88" distance of L14 L20
  measures "d89" distance of L15 L17
  measures "d90" distance of L3 L27
  measures "d91" distance of L28.start L28.end
  measures "d92" distance of L28.start L30.end
  measures "d93" distance of L32.start L32.end
  measures "d94" distance of L32.start L34.end
  measures "d95" distance of L36.start L36.end
  measures "d96" distance of L36.start L38.end
  measures "d97" distance of L40.start L40.end
  measures "d98" distance of L40.start L42.end
  measures "d99" distance of L3 L31
  measures "d100" distance of L24 L30
  measures "d101" distance of L29 L39
  measures "d102" distance of L16 L38
  measures "d103" distance of L37 L43
  measures "d104" distance of L12 L42
  measures "d105" distance of L21 L35
  measures "d106" distance of L0 L34
  measures "d107" distance of L44.start L44.end
  measures "d108" distance of L44.start L46.end
  measures "d109" distance of L32 L46
  measures "d110" distance of L13 L47
  measures "d111" distance of L48.start L48.end
  measures "d112" distance of L48.start L50.end
  measures "d115" distance of L41 L51
  measures "d116" distance of L44 L50
extrude "Extrude19" cut sketch "Sketch6" against normal blind 1.2 contours L4 L5 L6 L7 | L8 L9 L10 L11 | L12 L13 L14 L15 | L16 L17 L18 L19 | L20 L21 L22 L23 | L24 L25 L26 L27 | L28 L29 L30 L31 | L32 L33 L34 L35 | L36 L37 L38 L39 | L40 L41 L42 L43 | L44 L45 L46 L47 | L48 L49 L50 L51
